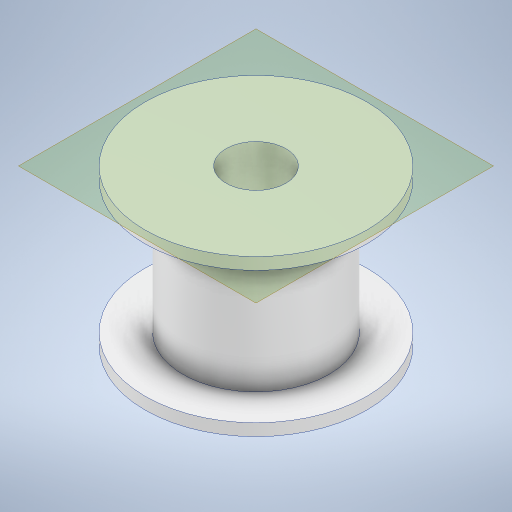
# Autodesk Inventor part: Idler Pulley 10mm 5mm Bore
Saved by Autodesk Inventor 2023 (Build 270158000, 158)
## iProperties
Created: 2023-12-10
Part Number: Idler Pulley 10mm 5mm Bore
Material: Aluminum 6061
Document SubType Name: Modeling
Designer: juanp
Density: 2.7 g/cm^3
Appearance: Aluminum - Flat
Author: juanp
Autodesk Inventor part; units mm, degrees
ref_plane "YZ Plane" through (0, 0, 0) normal (1, 0, 0) x (0, 1, 0)
ref_plane "XZ Plane" through (0, 0, 0) normal (0, 1, 0) x (-1, 0, 0)
ref_plane "XY Plane" through (0, 0, 0) normal (0, 0, 1) x (1, 0, 0)
sketch "Sketch1" plane through (0, 0, 0) normal (0, 1, 0) x (-1, 0, 0)
  circle A0 centre (0, 0) radius 9.25
  circle A1 centre (0, 0) radius 2.5
  circle A2 centre (0, 0) radius 6.1
  dimension "d0" = 18.5
  dimension "d1" = 5
  dimension "d4" = 12.2
  constraints: 3 centre point, 3 coincident
  measures "d0" diameter of A0
  measures "d1" diameter of A1
  measures "d4" diameter of A2
extrude "Extrusion1" add sketch "Sketch1" along normal blind 1 contours A0 | A2
ref_plane "Work Plane1" through (0, 13, 0) normal (0, -1, 0) x (1, 0, 0)
sketch "Sketch2" plane through (0, 13, 0) normal (0, -1, 0) x (1, 0, 0)
  circle A0 centre (0, 0) radius 9.25 projected
  circle A1 centre (0, 0) radius 2.5 projected
extrude "Extrusion2" add sketch "Sketch2" along normal blind 1
extrude "Extrusion3" add sketch "Sketch1" along normal up to surface (12 mm away) contours A2
body "Solid1"
